Autodesk Fusion 360 part; units mm, degrees
(part 8 of 11)
  line L3162 (205.13, 80.0836) -> (204.329, 80.0836)
  line L3163 (43.205, 99.7592) -> (42.406, 99.7592)
  line L3164 (-9.983, 10.9337) -> (-9.183, 10.9337)
  line L3165 (247.333, 38.5083) -> (247.929, 38.5083)
  line L3166 (-9.183, 14.0343) -> (-9.983, 14.0343)
  line L3167 (-28.52, 61.0336) -> (-28.52, 62.034)
  line L3168 (252.529, 29.4092) -> (252.529, 30.2332)
  line L3169 (205.13, 71.1844) -> (205.13, 76.9844)
  line L3170 (-143.3331, 10.9337) -> (-143.3331, 14.0343)
  line L3171 (200.082, 80.0836) -> (200.879, 80.0836)
  line L3172 (204.329, 68.0838) -> (205.13, 68.0838)
  line L3173 (42.406, 105.5592) -> (42.406, 108.6602)
  line L3174 (-9.983, 10.9337) -> (-9.983, 14.0343)
  line L3175 (-114.244, 105.5592) -> (-113.445, 105.5592)
  line L3176 (-22.957, 33.0844) -> (-23.758, 33.0844)
  line L3177 (43.205, 108.6602) -> (43.205, 109.6602)
  line L3178 (256.681, 31.9583) -> (255.761, 31.9583)
  line L3179 (-140.9519, 0.7845) -> (-140.1512, 0.7845)
  line L3180 (-14.233, 10.9337) -> (-13.432, 10.9337)
  line L3181 (-140.1512, 0.7845) -> (-140.1512, -5.0157)
  line L3182 (-28.52, 48.0333) -> (-28.52, 49.0338)
  line L3183 (243.459, 30.2332) -> (249.732, 30.2332)
  line L3184 (-140.9519, -5.0157) -> (-140.9519, -8.1163)
  line L3185 (-23.758, 41.9836) -> (-23.758, 42.984)
  line L3186 (200.879, 80.0836) -> (200.879, 76.9844)
  line L3187 (-140.9519, 0.7845) -> (-140.9519, 3.8837)
  line L3188 (200.879, 68.0838) -> (200.082, 68.0838)
  line L3189 (-142.5325, 9.9333) -> (-142.5325, 10.9337)
  line L3190 (255.761, 31.9583) -> (255.761, 30.2332)
  line L3191 (249.732, 30.2332) -> (243.459, 30.2332)
  line L3192 (249.732, 30.2332) -> (249.732, 29.4092)
  line L3193 (205.13, 76.9844) -> (205.13, 71.1844)
  line L3194 (200.082, 81.084) -> (186.08, 81.084)
  line L3195 (200.082, 67.0833) -> (186.08, 67.0833)
  line L3196 (5.618, 10.9337) -> (4.817, 10.9337)
  line L3197 (-18.708, 41.9836) -> (-19.508, 41.9836)
  line L3198 (200.082, 71.1844) -> (200.879, 71.1844)
  line L3199 (7.398, -18.7426) -> (7.398, -15.9426)
  line L3200 (-140.9519, -5.0157) -> (-140.1512, -5.0157)
  line L3201 (-142.5325, 14.0343) -> (-143.3331, 14.0343)
  line L3202 (-143.3331, 14.0343) -> (-142.5325, 14.0343)
  line L3203 (43.205, 96.6592) -> (42.406, 96.6592)
  line L3204 (-27.72, 52.1344) -> (-28.52, 52.1344)
  line L3205 (-143.3331, 14.0343) -> (-143.3331, 10.9337)
  line L3206 (-143.3331, 10.9337) -> (-142.5325, 10.9337)
  line L3207 (4.817, 9.9333) -> (4.817, 10.9337)
  line L3208 (-18.708, 42.984) -> (-18.708, 41.9836)
  line L3209 (-18.708, 33.0844) -> (-19.508, 33.0844)
  line L3210 (9.581, 61.0336) -> (9.581, 62.034)
  line L3211 (-142.5325, 10.9337) -> (-143.3331, 10.9337)
  line L3212 (-13.432, 10.9337) -> (-14.233, 10.9337)
  line L3213 (-28.52, 61.0336) -> (-27.72, 61.0336)
  line L3214 (-18.708, 33.0844) -> (-18.708, 38.8844)
  line L3215 (4.817, 10.9337) -> (4.817, 9.9333)
  line L3216 (186.08, 81.084) -> (200.082, 81.084)
  line L3217 (42.406, 105.5592) -> (43.205, 105.5592)
  line L3218 (43.205, 96.6592) -> (43.205, 95.6582)
  line L3219 (-28.52, 52.1344) -> (-27.72, 52.1344)
  line L3220 (-27.72, 57.9344) -> (-28.52, 57.9344)
  line L3221 (-23.758, 33.0844) -> (-22.957, 33.0844)
  line L3222 (43.205, 109.6602) -> (43.205, 108.6602)
  line L3223 (186.08, 67.0833) -> (200.082, 67.0833)
  line L3224 (-114.758, 41.9836) -> (-114.758, 38.8844)
  line L3225 (-23.758, 38.8844) -> (-23.758, 33.0844)
  line L3226 (-140.9519, -8.1163) -> (-140.1512, -8.1163)
  line L3227 (-113.9576, 41.9836) -> (-114.758, 41.9836)
  line L3228 (9.867, 19.8345) -> (9.867, 14.0343)
  line L3229 (-44.901, 0.1836) -> (-84.5267, 0.1836)
  line L3230 (-28.52, 57.9344) -> (-27.72, 57.9344)
  line L3231 (28.798, 120.9832) -> (9.398, 120.9832)
  line L3232 (43.205, 108.6602) -> (42.406, 108.6602)
  line L3233 (42.406, 96.6592) -> (42.406, 99.7592)
  line L3234 (238.182, 62.034) -> (224.18, 62.034)
  line L3235 (-19.508, 38.8844) -> (-19.508, 41.9836)
  line L3236 (-28.52, 48.0333) -> (-42.52, 48.0333)
  line L3237 (-137.77, 48.0333) -> (-137.77, 49.0338)
  line L3238 (10.38, 49.0338) -> (10.38, 52.1344)
  line L3239 (9.581, 57.9344) -> (9.581, 52.1344)
  line L3240 (-13.432, 14.0343) -> (-13.432, 10.9337)
  line L3241 (-9.183, 9.9333) -> (-9.183, 10.9337)
  line L3242 (-9.183, 10.9337) -> (-9.983, 10.9337)
  line L3243 (14.63, 57.9344) -> (14.63, 52.1344)
  line L3244 (-14.233, 9.9333) -> (-14.233, 10.9337)
  line L3245 (-22.957, 41.9836) -> (-22.957, 38.8844)
  line L3246 (-23.758, 38.8844) -> (-22.957, 38.8844)
  line L3247 (-66.333, 23.934) -> (-52.333, 23.934)
  line L3248 (-137.77, 57.9344) -> (-138.5693, 57.9344)
  line L3249 (242.482, 55.7585) -> (242.482, 59.0591)
  line L3250 (-118.2075, 38.8844) -> (-118.2075, 41.9836)
  line L3251 (-42.52, 48.0333) -> (-28.52, 48.0333)
  line L3252 (-140.1512, 0.7845) -> (-140.9519, 0.7845)
  line L3253 (-23.758, 33.0844) -> (-23.758, 38.8844)
  line L3254 (-113.9576, 42.984) -> (-113.9576, 41.9836)
  line L3255 (-114.758, 33.0844) -> (-113.9576, 33.0844)
  line L3256 (43.205, 95.6582) -> (43.205, 96.6592)
  line L3257 (-138.5693, 57.9344) -> (-138.5693, 61.0336)
  line L3258 (19.106, 81.084) -> (5.105, 81.084)
  arc A55 (7.398, -18.7426) -> (9.398, -20.7426) centre (9.398, -18.7426) ccw
  line L3259 (-137.77, 62.034) -> (-137.77, 61.0336)
  line L3260 (-18.708, 38.8844) -> (-18.708, 33.0844)
  line L3261 (-149.9629, 14.0343) -> (-149.9629, 19.8345)
  line L3262 (-42.52, 62.034) -> (-28.52, 62.034)
  line L3263 (42.406, 99.7592) -> (42.406, 96.6592)
  line L3264 (-114.758, 38.8844) -> (-114.758, 41.9836)
  line L3265 (-57.094, 99.7592) -> (-57.094, 105.5592)
  line L3266 (42.406, 99.7592) -> (43.205, 99.7592)
  line L3267 (-138.5693, 57.9344) -> (-137.77, 57.9344)
  line L3268 (255.761, 60.7841) -> (252.529, 60.7841)
  line L3269 (-27.72, 49.0338) -> (-28.52, 49.0338)
  line L3270 (-19.508, 38.8844) -> (-18.708, 38.8844)
  line L3271 (9.398, -20.7426) -> (28.798, -20.7426)
  line L3272 (-138.5693, 52.1344) -> (-137.77, 52.1344)
  line L3273 (249.732, 61.6082) -> (249.732, 60.7841)
  line L3274 (-56.295, 99.7592) -> (-57.094, 99.7592)
  line L3275 (-113.9576, 33.0844) -> (-114.758, 33.0844)
  line L3276 (9.867, 9.9333) -> (23.867, 9.9333)
  line L3277 (-56.295, 96.6592) -> (-56.295, 99.7592)
  line L3278 (-118.2075, 41.9836) -> (-118.2075, 38.8844)
  line L3279 (43.205, 99.7592) -> (43.205, 105.5592)
  line L3280 (-27.72, 61.0336) -> (-28.52, 61.0336)
  line L3281 (249.732, 60.7841) -> (243.459, 60.7841)
  line L3282 (4.817, 14.0343) -> (4.817, 19.8345)
  line L3283 (-23.758, 42.984) -> (-23.758, 41.9836)
  line L3284 (42.406, 108.6602) -> (42.406, 105.5592)
  line L3285 (-28.52, 62.034) -> (-42.52, 62.034)
  line L3286 (-19.508, 41.9836) -> (-19.508, 38.8844)
  line L3287 (-137.77, 52.1344) -> (-137.77, 57.9344)
  line L3288 (238.182, 22.9336) -> (238.182, 23.934)
  line L3289 (238.182, 61.0336) -> (238.182, 62.034)
  line L3290 (23.867, 14.0343) -> (23.867, 19.8345)
  line L3291 (23.867, 9.9333) -> (9.867, 9.9333)
  line L3292 (43.205, 105.5592) -> (43.205, 99.7592)
  line L3293 (-28.52, 49.0338) -> (-27.72, 49.0338)
  line L3294 (-22.957, 38.8844) -> (-22.957, 41.9836)
  line L3295 (-114.244, 95.6582) -> (-128.2451, 95.6582)
  line L3296 (-19.508, 33.0844) -> (-18.708, 33.0844)
  line L3297 (-28.52, 57.9344) -> (-28.52, 52.1344)
  line L3298 (-57.094, 108.6602) -> (-56.295, 108.6602)
  line L3299 (-137.77, 61.0336) -> (-138.5693, 61.0336)
  line L3300 (-19.508, 41.9836) -> (-18.708, 41.9836)
  line L3301 (-57.094, 108.6602) -> (-57.094, 109.6602)
  line L3302 (-113.9576, 29.9838) -> (-113.9576, 28.9833)
  line L3303 (-137.77, 49.0338) -> (-138.5693, 49.0338)
  line L3304 (28.917, 19.8345) -> (28.917, 14.0343)
  line L3305 (-57.094, 95.6582) -> (-57.094, 96.6592)
  line L3306 (-14.233, 14.0343) -> (-14.233, 19.8345)
  line L3307 (-57.094, 96.6592) -> (-57.094, 95.6582)
  line L3308 (242.482, 20.959) -> (243.459, 20.959)
  line L3309 (43.205, 105.5592) -> (42.406, 105.5592)
  line L3310 (-56.295, 105.5592) -> (-57.094, 105.5592)
  line L3311 (-28.52, 52.1344) -> (-28.52, 57.9344)
  line L3312 (-22.957, 41.9836) -> (-23.758, 41.9836)
  line L3313 (-22.957, 38.8844) -> (-23.758, 38.8844)
  line L3314 (242.482, 59.0591) -> (243.459, 59.0591)
  line L3315 (42.406, 108.6602) -> (43.205, 108.6602)
  line L3316 (256.681, 59.0591) -> (255.761, 59.0591)
  line L3317 (-52.045, 67.0833) -> (-38.044, 67.0833)
  line L3318 (252.529, 22.6841) -> (255.761, 22.6841)
  line L3319 (-118.2075, 33.0844) -> (-118.2075, 29.9838)
  line L3320 (-113.9576, 29.9838) -> (-114.758, 29.9838)
  line L3321 (-137.77, 57.9344) -> (-137.77, 52.1344)
  line L3322 (238.979, 57.9344) -> (238.182, 57.9344)
  line L3323 (-14.233, 19.8345) -> (-14.233, 14.0343)
  line L3324 (243.459, 22.6841) -> (249.732, 22.6841)
  line L3325 (-114.758, 29.9838) -> (-114.758, 33.0844)
  line L3326 (-28.52, 62.034) -> (-28.52, 61.0336)
  line L3327 (-138.5693, 52.1344) -> (-138.5693, 49.0338)
  line L3328 (238.979, 61.0336) -> (238.979, 57.9344)
  line L3329 (-137.77, 61.0336) -> (-137.77, 62.034)
  line L3330 (4.817, 19.8345) -> (4.817, 14.0343)
  line L3331 (-114.758, 33.0844) -> (-114.758, 29.9838)
  line L3332 (-138.5693, 49.0338) -> (-138.5693, 52.1344)
  line L3333 (252.529, 60.7841) -> (252.529, 61.6082)
  line L3334 (-18.708, 41.9836) -> (-18.708, 42.984)
  line L3335 (249.732, 22.6841) -> (243.459, 22.6841)
  line L3336 (-143.2635, 114.1832) -> (-108.601, 114.1832)
  line L3337 (-57.094, 109.6602) -> (-57.094, 108.6602)
  line L3338 (-9.183, 14.0343) -> (-9.183, 19.8345)
  line L3339 (-163.9637, 19.8345) -> (-163.9637, 14.0343)
  line L3340 (-56.295, 105.5592) -> (-56.295, 108.6602)
  line L3341 (-113.9576, 38.8844) -> (-114.758, 38.8844)
  line L3342 (-137.77, 49.0338) -> (-137.77, 48.0333)
  line L3343 (28.917, 14.0343) -> (28.917, 19.8345)
  line L3344 (238.979, 19.8345) -> (238.182, 19.8345)
  line L3345 (-57.094, 105.5592) -> (-56.295, 105.5592)
  line L3346 (-149.9629, 9.9333) -> (-149.9629, 10.9337)
  line L3347 (42.917, 19.8345) -> (42.917, 14.0343)
  line L3348 (-114.758, 41.9836) -> (-113.9576, 41.9836)
  line L3349 (-9.183, 19.8345) -> (-9.183, 14.0343)
  line L3350 (249.732, 60.7841) -> (249.732, 61.6082)
  line L3351 (-23.758, 41.9836) -> (-22.957, 41.9836)
  line L3352 (-113.9576, 41.9836) -> (-113.9576, 42.984)
  line L3353 (-18.708, 38.8844) -> (-19.508, 38.8844)
  line L3354 (238.182, 19.8345) -> (238.979, 19.8345)
  line L3355 (238.182, 57.9344) -> (238.979, 57.9344)
  line L3356 (-57.094, 105.5592) -> (-57.094, 99.7592)
  line L3357 (-163.9637, 9.9333) -> (-163.9637, 10.9337)
  line L3358 (-138.5693, 61.0336) -> (-138.5693, 57.9344)
  line L3359 (-138.5693, 49.0338) -> (-137.77, 49.0338)
  line L3360 (9.867, 14.0343) -> (9.867, 19.8345)
  line L3361 (256.681, 20.959) -> (256.681, 17.6585)
  line L3362 (14.63, 49.0338) -> (13.831, 49.0338)
  line L3363 (252.529, 60.7841) -> (255.761, 60.7841)
  line L3364 (-118.2075, 29.9838) -> (-118.2075, 33.0844)
  line L3365 (238.182, 22.9336) -> (238.979, 22.9336)
  line L3366 (-57.094, 96.6592) -> (-56.295, 96.6592)
  line L3367 (-163.9637, 3.8837) -> (-163.9637, 4.8841)
  line L3368 (255.761, 20.959) -> (256.681, 20.959)
  line L3369 (-164.763, 14.0343) -> (-163.9637, 14.0343)
  line L3370 (42.917, 14.0343) -> (42.917, 19.8345)
  line L3371 (-138.5693, 61.0336) -> (-137.77, 61.0336)
  line L3372 (255.761, 20.959) -> (255.761, 22.6841)
  line L3373 (-56.295, 99.7592) -> (-56.295, 96.6592)
  line L3374 (255.761, 59.0591) -> (255.761, 60.7841)
  line L3375 (9.581, 52.1344) -> (10.38, 52.1344)
  line L3376 (-114.758, 29.9838) -> (-113.9576, 29.9838)
  line L3377 (-137.77, 52.1344) -> (-138.5693, 52.1344)
  line L3378 (-114.758, 38.8844) -> (-113.9576, 38.8844)
  line L3379 (243.459, 60.7841) -> (249.732, 60.7841)
  line L3380 (255.761, 59.0591) -> (256.681, 59.0591)
  line L3381 (-113.9576, 38.8844) -> (-113.9576, 33.0844)
  line L3382 (-163.9637, 4.8841) -> (-163.9637, 3.8837)
  line L3383 (-56.295, 108.6602) -> (-56.295, 105.5592)
  line L3384 (-142.5325, 14.0343) -> (-142.5325, 19.8345)
  line L3385 (10.38, 61.0336) -> (9.581, 61.0336)
  line L3386 (-29.033, 19.8345) -> (-28.233, 19.8345)
  line L3387 (13.831, 49.0338) -> (14.63, 49.0338)
  line L3388 (-56.295, 108.6602) -> (-57.094, 108.6602)
  line L3389 (255.761, 22.6841) -> (255.761, 20.959)
  line L3390 (-119.0079, 29.9838) -> (-118.2075, 29.9838)
  line L3391 (13.831, 52.1344) -> (13.831, 49.0338)
  line L3392 (-118.2075, 33.0844) -> (-119.0079, 33.0844)
  line L3393 (-164.763, 3.8837) -> (-163.9637, 3.8837)
  line L3394 (242.482, 59.0591) -> (242.482, 55.7585)
  line L3395 (-56.295, 96.6592) -> (-57.094, 96.6592)
  line L3396 (243.459, 59.0591) -> (242.482, 59.0591)
  line L3397 (13.831, 99.7592) -> (13.831, 96.6592)
  line L3398 (-113.9576, 28.9833) -> (-113.9576, 29.9838)
  line L3399 (14.63, 99.7592) -> (13.831, 99.7592)
  line L3400 (-57.094, 99.7592) -> (-56.295, 99.7592)
  line L3401 (242.482, 20.959) -> (242.482, 17.6585)
  line L3402 (-149.9629, 3.8837) -> (-149.1636, 3.8837)
  line L3403 (238.182, 67.0833) -> (224.18, 67.0833)
  line L3404 (-32.995, 67.0833) -> (-32.995, 68.0838)
  line L3405 (-113.9576, 33.0844) -> (-113.9576, 38.8844)
  line L3406 (-164.763, 10.9337) -> (-163.9637, 10.9337)
  line L3407 (-163.9637, 9.9333) -> (-149.9629, 9.9333)
  line L3408 (243.459, 20.959) -> (243.459, 22.6841)
  line L3409 (242.482, 17.6585) -> (242.482, 20.959)
  line L3410 (-4.42, 95.6582) -> (9.581, 95.6582)
  line L3411 (-33.794, 80.0836) -> (-32.995, 80.0836)
  line L3412 (238.979, 57.9344) -> (238.979, 61.0336)
  line L3413 (-33.794, 76.9844) -> (-33.794, 80.0836)
  line L3414 (252.529, 61.6082) -> (252.529, 60.7841)
  line L3415 (-28.233, 22.9336) -> (-29.033, 22.9336)
  line L3416 (9.581, 52.1344) -> (9.581, 57.9344)
  line L3417 (-32.995, 68.0838) -> (-32.995, 67.0833)
  line L3418 (28.631, 99.7592) -> (29.43, 99.7592)
  line L3419 (28.631, 96.6592) -> (29.43, 96.6592)
  line L3420 (256.681, 20.959) -> (255.761, 20.959)
  line L3421 (-33.794, 71.1844) -> (-32.995, 71.1844)
  line L3422 (238.182, 23.934) -> (238.182, 22.9336)
  line L3423 (9.581, 105.5592) -> (9.581, 99.7592)
  line L3424 (14.63, 61.0336) -> (14.63, 62.034)
  line L3425 (29.43, 96.6592) -> (28.631, 96.6592)
  line L3426 (-118.2075, 29.9838) -> (-119.0079, 29.9838)
  line L3427 (-32.995, 76.9844) -> (-32.995, 71.1844)
  line L3428 (-119.0079, 41.9836) -> (-119.0079, 42.984)
  line L3429 (14.63, 96.6592) -> (14.63, 95.6582)
  line L3430 (249.732, 22.6841) -> (249.732, 23.5082)
  line L3431 (-119.0079, 38.8844) -> (-119.0079, 33.0844)
  line L3432 (-163.9637, 10.9337) -> (-163.9637, 9.9333)
  line L3433 (-149.9629, 14.0343) -> (-149.1636, 14.0343)
  line L3434 (10.38, 61.0336) -> (10.38, 57.9344)
  line L3435 (243.459, 59.0591) -> (243.459, 60.7841)
  line L3436 (238.182, 62.034) -> (238.182, 61.0336)
  line L3437 (-33.794, 68.0838) -> (-33.794, 71.1844)
  line L3438 (9.581, 96.6592) -> (9.581, 95.6582)
  line L3439 (-149.9629, 3.8837) -> (-149.9629, 4.8841)
  line L3440 (-28.233, 19.8345) -> (-29.033, 19.8345)
  line L3441 (-33.794, 76.9844) -> (-32.995, 76.9844)
  line L3442 (-18.708, 29.9838) -> (-18.708, 28.9833)
  line L3443 (-71.8941, 96.6592) -> (-71.8941, 99.7592)
  line L3444 (-71.8941, 108.6602) -> (-71.8941, 105.5592)
  line L3445 (255.761, 22.6841) -> (252.529, 22.6841)
  line L3446 (-71.8941, 99.7592) -> (-71.8941, 96.6592)
  line L3447 (-149.1636, 3.8837) -> (-149.9629, 3.8837)
  line L3448 (252.529, 61.6082) -> (249.732, 61.6082)
  line L3449 (243.459, 60.7841) -> (243.459, 59.0591)
  line L3450 (-23.758, 29.9838) -> (-22.957, 29.9838)
  line L3451 (14.63, 57.9344) -> (13.831, 57.9344)
  line L3452 (13.831, 96.6592) -> (14.63, 96.6592)
  line L3453 (-118.2075, 38.8844) -> (-119.0079, 38.8844)
  line L3454 (10.38, 99.7592) -> (9.581, 99.7592)
  line L3455 (14.63, 61.0336) -> (13.831, 61.0336)
  line L3456 (14.63, 95.6582) -> (14.63, 96.6592)
  line L3457 (-23.758, 28.9833) -> (-23.758, 29.9838)
  line L3458 (-33.794, 80.0836) -> (-33.794, 76.9844)
  line L3459 (-71.8941, 105.5592) -> (-71.8941, 108.6602)
  line L3460 (249.732, 23.5082) -> (249.732, 22.6841)
  line L3461 (-29.033, 22.9336) -> (-29.033, 19.8345)
  line L3462 (-28.233, 22.9336) -> (-28.233, 23.934)
  line L3463 (29.43, 99.7592) -> (29.43, 96.6592)
  line L3464 (-164.763, 14.0343) -> (-164.763, 10.9337)
  line L3465 (28.631, 96.6592) -> (28.631, 95.6582)
  line L3466 (238.979, 61.0336) -> (238.182, 61.0336)
  line L3467 (-32.995, 80.0836) -> (-32.995, 81.084)
  line L3468 (-57.094, 109.6602) -> (-71.095, 109.6602)
  line L3469 (9.581, 109.6602) -> (9.581, 108.6602)
  line L3470 (-75.345, 108.6602) -> (-76.144, 108.6602)
  line L3471 (13.831, 49.0338) -> (13.831, 52.1344)
  line L3472 (-149.1636, 10.9337) -> (-149.9629, 10.9337)
  line L3473 (9.581, 108.6602) -> (10.38, 108.6602)
  line L3474 (-149.9629, 4.8841) -> (-149.9629, 3.8837)
  line L3475 (238.979, 22.9336) -> (238.979, 19.8345)
  line L3476 (256.681, 55.7585) -> (256.681, 59.0591)
  line L3477 (243.459, 22.6841) -> (243.459, 20.959)
  line L3478 (-119.0079, 28.9833) -> (-119.0079, 29.9838)
  line L3479 (-71.8941, 108.6602) -> (-71.095, 108.6602)
  line L3480 (-32.995, 81.084) -> (-32.995, 80.0836)
  line L3481 (-119.0079, 33.0844) -> (-119.0079, 38.8844)
  line L3482 (255.761, 60.7841) -> (255.761, 59.0591)
  line L3483 (14.63, 62.034) -> (14.63, 61.0336)
  line L3484 (-119.0079, 42.984) -> (-119.0079, 41.9836)
  line L3485 (-163.9637, 3.8837) -> (-164.763, 3.8837)
  line L3486 (-71.8941, 99.7592) -> (-71.095, 99.7592)
  line L3487 (-33.794, 68.0838) -> (-32.995, 68.0838)
  line L3488 (-83.201, 118.9832) -> (-83.201, 116.1832)
  line L3489 (-119.0079, 38.8844) -> (-118.2075, 38.8844)
  line L3490 (-32.995, 68.0838) -> (-33.794, 68.0838)
  line L3491 (9.581, 49.0338) -> (9.581, 48.0333)
  line L3492 (10.38, 96.6592) -> (10.38, 99.7592)
  line L3493 (-32.995, 80.0836) -> (-33.794, 80.0836)
  line L3494 (-71.095, 105.5592) -> (-71.8941, 105.5592)
  line L3495 (256.681, 59.0591) -> (256.681, 55.7585)
  line L3496 (238.979, 22.9336) -> (238.182, 22.9336)
  line L3497 (-22.957, 29.9838) -> (-23.758, 29.9838)
  line L3498 (9.581, 99.7592) -> (9.581, 105.5592)
  line L3499 (-71.095, 109.6602) -> (-71.095, 108.6602)
  line L3500 (-75.345, 99.7592) -> (-76.144, 99.7592)
  line L3501 (-119.0079, 29.9838) -> (-119.0079, 28.9833)
  line L3502 (10.38, 57.9344) -> (10.38, 61.0336)
  line L3503 (249.732, 61.6082) -> (252.529, 61.6082)
  line L3504 (-119.0079, 33.0844) -> (-118.2075, 33.0844)
  line L3505 (-76.144, 99.7592) -> (-75.345, 99.7592)
  line L3506 (14.63, 95.6582) -> (28.631, 95.6582)
  line L3507 (28.631, 95.6582) -> (14.63, 95.6582)
  line L3508 (10.38, 96.6592) -> (9.581, 96.6592)
  line L3509 (-18.708, 29.9838) -> (-19.508, 29.9838)
  line L3510 (-163.9637, 4.8841) -> (-149.9629, 4.8841)
  line L3511 (28.631, 95.6582) -> (28.631, 96.6592)
  line L3512 (-23.758, 29.9838) -> (-23.758, 28.9833)
  line L3513 (249.732, 23.5082) -> (252.529, 23.5082)
  line L3514 (-149.9629, 4.8841) -> (-163.9637, 4.8841)
  line L3515 (-128.2451, 71.1844) -> (-129.0441, 71.1844)
  line L3516 (-29.033, 22.9336) -> (-28.233, 22.9336)
  line L3517 (238.979, 19.8345) -> (238.979, 22.9336)
  line L3518 (-32.995, 71.1844) -> (-33.794, 71.1844)
  line L3519 (-118.2075, 41.9836) -> (-119.0079, 41.9836)
  line L3520 (-132.495, 76.9844) -> (-133.294, 76.9844)
  line L3521 (252.529, 22.6841) -> (252.529, 23.5082)
  line L3522 (-32.995, 71.1844) -> (-32.995, 76.9844)
  line L3523 (-32.995, 76.9844) -> (-33.794, 76.9844)
  line L3524 (-132.495, 68.0838) -> (-133.294, 68.0838)
  line L3525 (-71.095, 96.6592) -> (-71.8941, 96.6592)
  line L3526 (10.38, 99.7592) -> (10.38, 96.6592)
  line L3527 (-28.233, 23.934) -> (-28.233, 22.9336)
  line L3528 (13.831, 99.7592) -> (14.63, 99.7592)
  arc A56 (9.398, 120.9832) -> (7.398, 118.9832) centre (9.398, 118.9832) ccw
  line L3529 (-76.144, 105.5592) -> (-76.144, 99.7592)
  line L3530 (-71.8941, 96.6592) -> (-71.095, 96.6592)
  line L3531 (13.831, 96.6592) -> (13.831, 99.7592)
  line L3532 (238.182, 61.0336) -> (238.979, 61.0336)
  line L3533 (9.581, 105.5592) -> (10.38, 105.5592)
  line L3534 (-19.508, 29.9838) -> (-18.708, 29.9838)
  line L3535 (9.581, 108.6602) -> (9.581, 109.6602)
  line L3536 (29.43, 99.7592) -> (28.631, 99.7592)
  line L3537 (-132.495, 80.0836) -> (-132.495, 76.9844)
  line L3538 (-76.144, 108.6602) -> (-75.345, 108.6602)
  line L3539 (-76.144, 96.6592) -> (-76.144, 95.6582)
  line L3540 (-18.708, 28.9833) -> (-18.708, 29.9838)
  line L3541 (-149.1636, 14.0343) -> (-149.9629, 14.0343)
  line L3542 (-149.9629, 9.9333) -> (-163.9637, 9.9333)
  line L3543 (-149.1636, 10.9337) -> (-149.1636, 14.0343)
  line L3544 (-71.095, 95.6582) -> (-57.094, 95.6582)
  line L3545 (-119.0079, 41.9836) -> (-118.2075, 41.9836)
  line L3546 (256.681, 17.6585) -> (256.681, 20.959)
  line L3547 (29.43, 96.6592) -> (29.43, 99.7592)
  line L3548 (-147.583, 57.9344) -> (-147.583, 52.1344)
  line L3549 (-5.219, 49.0338) -> (-5.219, 52.1344)
  line L3550 (-42.007, 29.9838) -> (-42.007, 33.0844)
  line L3551 (256.23, 15.2084) -> (256.23, 14.4091)
  line L3552 (-42.808, 41.9836) -> (-42.007, 41.9836)
  line L3553 (-9.469, 109.6602) -> (-9.469, 108.6602)
  line L3554 (-104.4326, 9.9333) -> (-104.4326, 10.9337)
  line L3555 (-8.67, 49.0338) -> (-8.67, 52.1344)
  line L3556 (-9.469, 49.0338) -> (-9.469, 48.0333)
  line L3557 (247.929, -1.1159) -> (243.459, -1.1159)
  line L3558 (238.182, -9.1167) -> (238.182, -8.1163)
  line L3559 (253.129, 14.4091) -> (252.529, 14.4091)
  line L3560 (-8.67, 108.6602) -> (-9.469, 108.6602)
  line L3561 (-4.42, 57.9344) -> (-4.42, 52.1344)
  line L3562 (-4.42, 61.0336) -> (-5.219, 61.0336)
  line L3563 (-105.233, 10.9337) -> (-104.4326, 10.9337)
  line L3564 (255.761, 17.6585) -> (256.681, 17.6585)
  line L3565 (-9.469, 108.6602) -> (-8.67, 108.6602)
  line L3566 (-9.469, 99.7592) -> (-9.469, 105.5592)
  line L3567 (-4.42, 109.6602) -> (9.581, 109.6602)
  line L3568 (249.732, -7.8669) -> (243.459, -7.8669)
  line L3569 (243.459, -7.8669) -> (249.732, -7.8669)
  line L3570 (-61.57, 52.1344) -> (-62.371, 52.1344)
  line L3571 (238.979, 0.7845) -> (238.979, 3.8837)
  line L3572 (-37.758, 33.0844) -> (-37.758, 38.8844)
  line L3573 (-9.469, 49.0338) -> (-8.67, 49.0338)
  line L3574 (-147.583, 61.0336) -> (-147.583, 62.034)
  line L3575 (-4.42, 62.034) -> (-4.42, 61.0336)
  line L3576 (-37.758, 29.9838) -> (-37.758, 28.9833)
  line L3577 (252.529, 15.9333) -> (252.529, 14.4091)
  line L3578 (-8.67, 52.1344) -> (-9.469, 52.1344)
  line L3579 (-147.583, 49.0338) -> (-146.7824, 49.0338)
  line L3580 (0.855, 80.0836) -> (0.056, 80.0836)
  line L3581 (255.761, 15.9333) -> (255.761, 17.6585)
  line L3582 (-9.469, 96.6592) -> (-8.67, 96.6592)
  line L3583 (-105.233, 14.0343) -> (-105.233, 10.9337)
  line L3584 (-8.67, 52.1344) -> (-8.67, 49.0338)
  line L3585 (238.182, -8.1163) -> (238.979, -8.1163)
  line L3586 (-146.7824, 49.0338) -> (-147.583, 49.0338)
  line L3587 (-5.219, 52.1344) -> (-4.42, 52.1344)
  line L3588 (-42.808, 29.9838) -> (-42.007, 29.9838)
  line L3589 (252.529, 14.4091) -> (252.529, 15.9333)
  line L3590 (-4.42, 57.9344) -> (-5.219, 57.9344)
  line L3591 (-8.67, 61.0336) -> (-8.67, 57.9344)
  line L3592 (-104.4326, 14.0343) -> (-104.4326, 19.8345)
  line L3593 (-42.808, 38.8844) -> (-42.007, 38.8844)
  line L3594 (-147.583, 49.0338) -> (-147.583, 48.0333)
  line L3595 (-129.0441, 105.5592) -> (-128.2451, 105.5592)
  line L3596 (253.129, 14.4091) -> (253.129, 15.2084)
  line L3597 (255.761, 17.6585) -> (255.761, 15.9333)
  line L3598 (4.306, 71.1844) -> (4.306, 68.0838)
  line L3599 (-9.469, 48.0333) -> (-9.469, 49.0338)
  line L3600 (238.182, 3.8837) -> (238.182, 4.8841)
  line L3601 (-9.469, 95.6582) -> (-9.469, 96.6592)
  line L3602 (238.182, 0.7845) -> (238.979, 0.7845)
  line L3603 (-104.4326, 10.9337) -> (-104.4326, 9.9333)
  line L3604 (-8.67, 99.7592) -> (-9.469, 99.7592)
  line L3605 (-42.808, 41.9836) -> (-42.808, 42.984)
  line L3606 (-109.4829, 19.8345) -> (-109.4829, 14.0343)
  line L3607 (-56.808, 28.9833) -> (-42.808, 28.9833)
  line L3608 (4.306, 76.9844) -> (4.306, 80.0836)
  line L3609 (-89.6325, 10.9337) -> (-90.4329, 10.9337)
  line L3610 (-8.67, 49.0338) -> (-9.469, 49.0338)
  line L3611 (-146.7824, 57.9344) -> (-147.583, 57.9344)
  line L3612 (-71.095, 99.7592) -> (-71.8941, 99.7592)
  line L3613 (-33.794, 71.1844) -> (-33.794, 68.0838)
  line L3614 (252.529, 23.5082) -> (252.529, 22.6841)
  line L3615 (-149.9629, 10.9337) -> (-149.1636, 10.9337)
  line L3616 (-132.495, 71.1844) -> (-132.495, 68.0838)
  line L3617 (243.459, 20.959) -> (242.482, 20.959)
  line L3618 (-19.508, 29.9838) -> (-19.508, 33.0844)
  line L3619 (-129.0441, 80.0836) -> (-128.2451, 80.0836)
  line L3620 (14.63, 96.6592) -> (13.831, 96.6592)
  line L3621 (-75.345, 99.7592) -> (-75.345, 96.6592)
  line L3622 (-164.763, 10.9337) -> (-164.763, 14.0343)
  line L3623 (-76.144, 96.6592) -> (-75.345, 96.6592)
  line L3624 (-132.495, 68.0838) -> (-132.495, 71.1844)
  line L3625 (-57.094, 95.6582) -> (-71.095, 95.6582)
  line L3626 (-19.508, 33.0844) -> (-19.508, 29.9838)
  line L3627 (-163.9637, 14.0343) -> (-164.763, 14.0343)
  line L3628 (-22.957, 29.9838) -> (-22.957, 33.0844)
  line L3629 (-133.294, 76.9844) -> (-132.495, 76.9844)
  arc A57 (5.398, 114.1832) -> (7.398, 116.1832) centre (5.398, 116.1832) ccw
  line L3630 (10.38, 105.5592) -> (9.581, 105.5592)
  line L3631 (9.581, 99.7592) -> (10.38, 99.7592)
  line L3632 (-128.2451, 81.084) -> (-128.2451, 80.0836)
  line L3633 (-71.095, 99.7592) -> (-71.095, 105.5592)
  line L3634 (-76.144, 95.6582) -> (-76.144, 96.6592)
  line L3635 (-76.144, 99.7592) -> (-76.144, 105.5592)
  line L3636 (7.398, 118.9832) -> (7.398, 116.1832)
  line L3637 (252.529, 23.5082) -> (249.732, 23.5082)
  line L3638 (-29.033, 19.8345) -> (-29.033, 22.9336)
  line L3639 (-163.9637, 10.9337) -> (-164.763, 10.9337)
  line L3640 (-71.095, 109.6602) -> (-57.094, 109.6602)
  line L3641 (10.38, 108.6602) -> (10.38, 105.5592)
  line L3642 (-76.144, 105.5592) -> (-75.345, 105.5592)
  line L3643 (-71.095, 108.6602) -> (-71.8941, 108.6602)
  line L3644 (19.905, 80.0836) -> (19.106, 80.0836)
  line L3645 (-75.345, 105.5592) -> (-76.144, 105.5592)
  line L3646 (-76.144, 109.6602) -> (-76.144, 108.6602)
  line L3647 (19.106, 80.0836) -> (19.905, 80.0836)
  line L3648 (10.38, 105.5592) -> (10.38, 108.6602)
  line L3649 (-71.8941, 105.5592) -> (-71.095, 105.5592)
  line L3650 (-129.0441, 68.0838) -> (-129.0441, 71.1844)
  line L3651 (242.429, 68.0838) -> (243.23, 68.0838)
  line L3652 (-149.9629, 10.9337) -> (-149.9629, 9.9333)
  line L3653 (-71.095, 95.6582) -> (-71.095, 96.6592)
  line L3654 (19.905, 71.1844) -> (19.106, 71.1844)
  line L3655 (19.106, 67.0833) -> (19.106, 68.0838)
  line L3656 (-133.294, 68.0838) -> (-133.294, 67.0833)
  line L3657 (-22.957, 33.0844) -> (-22.957, 29.9838)
  line L3658 (-75.345, 105.5592) -> (-75.345, 108.6602)
  line L3659 (238.182, 68.0838) -> (238.979, 68.0838)
  line L3660 (-129.0441, 71.1844) -> (-128.2451, 71.1844)
  line L3661 (-37.245, 76.9844) -> (-37.245, 80.0836)
  line L3662 (-75.345, 96.6592) -> (-76.144, 96.6592)
  line L3663 (-71.095, 105.5592) -> (-71.095, 99.7592)
  line L3664 (-38.044, 71.1844) -> (-38.044, 76.9844)
  line L3665 (-71.095, 96.6592) -> (-71.095, 95.6582)
  line L3666 (9.581, 96.6592) -> (10.38, 96.6592)
  line L3667 (9.581, 95.6582) -> (9.581, 96.6592)
  line L3668 (10.38, 108.6602) -> (9.581, 108.6602)
  line L3669 (-71.095, 108.6602) -> (-71.095, 109.6602)
  line L3670 (19.905, 68.0838) -> (19.905, 71.1844)
  line L3671 (238.979, 71.1844) -> (238.979, 68.0838)
  line L3672 (-133.294, 80.0836) -> (-133.294, 81.084)
  line L3673 (-149.1636, 14.0343) -> (-149.1636, 10.9337)
  line L3674 (-76.144, 108.6602) -> (-76.144, 109.6602)
  line L3675 (-132.495, 80.0836) -> (-133.294, 80.0836)
  line L3676 (258.029, 68.0838) -> (257.232, 68.0838)
  line L3677 (-128.5329, 19.8345) -> (-127.7325, 19.8345)
  line L3678 (-75.345, 108.6602) -> (-75.345, 105.5592)
  line L3679 (258.029, 68.0838) -> (258.029, 71.1844)
  line L3680 (-128.2451, 80.0836) -> (-129.0441, 80.0836)
  line L3681 (5.105, 67.0833) -> (19.106, 67.0833)
  line L3682 (-4.42, 48.0333) -> (9.581, 48.0333)
  line L3683 (257.232, 68.0838) -> (258.029, 68.0838)
  line L3684 (-38.044, 68.0838) -> (-37.245, 68.0838)
  line L3685 (-38.044, 71.1844) -> (-37.245, 71.1844)
  line L3686 (238.182, 42.984) -> (224.18, 42.984)
  line L3687 (-42.808, 28.9833) -> (-56.808, 28.9833)
  line L3688 (-38.044, 67.0833) -> (-38.044, 68.0838)
  line L3689 (19.106, 76.9844) -> (19.106, 71.1844)
  line L3690 (19.106, 68.0838) -> (19.905, 68.0838)
  line L3691 (-123.4826, 22.9336) -> (-124.283, 22.9336)
  arc A58 (-83.201, 116.1832) -> (-81.201, 114.1832) centre (-81.201, 116.1832) ccw
  line L3692 (19.106, 80.0836) -> (19.106, 81.084)
  line L3693 (224.18, 67.0833) -> (238.182, 67.0833)
  arc A59 (-83.201, 118.9832) -> (-85.201, 120.9832) centre (-85.201, 118.9832) ccw
  line L3694 (-38.044, 80.0836) -> (-38.044, 81.084)
  line L3695 (-129.0441, 76.9844) -> (-129.0441, 80.0836)
  line L3696 (243.23, 68.0838) -> (242.429, 68.0838)
  line L3697 (-38.044, 80.0836) -> (-37.245, 80.0836)
  line L3698 (-75.345, 96.6592) -> (-75.345, 99.7592)
  line L3699 (238.979, 71.1844) -> (238.182, 71.1844)
  line L3700 (19.905, 76.9844) -> (19.106, 76.9844)
  line L3701 (-4.42, 62.034) -> (9.581, 62.034)
  line L3702 (-37.245, 76.9844) -> (-38.044, 76.9844)
  line L3703 (-108.6825, 22.9336) -> (-109.4829, 22.9336)
  line L3704 (-104.4326, 19.8345) -> (-104.4326, 14.0343)
  line L3705 (19.106, 81.084) -> (19.106, 80.0836)
  line L3706 (14.63, 108.6602) -> (13.831, 108.6602)
  line L3707 (19.106, 76.9844) -> (19.905, 76.9844)
  line L3708 (243.23, 68.0838) -> (243.23, 67.0833)
  line L3709 (-128.5329, 22.9336) -> (-128.5329, 23.934)
  line L3710 (-133.294, 71.1844) -> (-132.495, 71.1844)
  line L3711 (-37.245, 68.0838) -> (-38.044, 68.0838)
  line L3712 (238.182, 67.0833) -> (238.182, 68.0838)
  line L3713 (28.631, 99.7592) -> (28.631, 105.5592)
  line L3714 (238.182, 71.1844) -> (238.979, 71.1844)
  line L3715 (13.831, 108.6602) -> (13.831, 105.5592)
  line L3716 (-149.1636, 0.7845) -> (-149.9629, 0.7845)
  line L3717 (-124.283, 22.9336) -> (-124.283, 19.8345)
  line L3718 (-38.044, 68.0838) -> (-38.044, 67.0833)
  circle A60 centre (19.098, 117.5832) radius 1.7
  line L3719 (-52.045, 81.084) -> (-38.044, 81.084)
  line L3720 (19.905, 76.9844) -> (19.905, 80.0836)
  line L3721 (247.333, 14.4091) -> (247.929, 14.4091)
  line L3722 (-149.9629, -9.1167) -> (-149.9629, -8.1163)
  line L3723 (-132.495, 76.9844) -> (-132.495, 80.0836)
  line L3724 (-133.294, 76.9844) -> (-133.294, 71.1844)
  line L3725 (-123.4826, 23.934) -> (-109.4829, 23.934)
  line L3726 (-123.769, 48.0333) -> (-137.77, 48.0333)
  line L3727 (247.333, 15.2084) -> (244.232, 15.2084)
  line L3728 (9.581, 62.034) -> (-4.42, 62.034)
  line L3729 (19.905, 71.1844) -> (19.905, 68.0838)
  line L3730 (238.979, 68.0838) -> (238.182, 68.0838)
  line L3731 (-128.5329, 22.9336) -> (-127.7325, 22.9336)
  line L3732 (224.18, 62.034) -> (238.182, 62.034)
  line L3733 (-37.245, 80.0836) -> (-38.044, 80.0836)
  line L3734 (19.106, 71.1844) -> (19.905, 71.1844)
  line L3735 (-129.0441, 80.0836) -> (-129.0441, 76.9844)
  line L3736 (28.631, 108.6602) -> (29.43, 108.6602)
  line L3737 (-109.4829, 23.934) -> (-123.4826, 23.934)
  line L3738 (-137.77, 48.0333) -> (-123.769, 48.0333)
  line L3739 (-164.763, -5.0157) -> (-164.763, -8.1163)
  line L3740 (19.905, 68.0838) -> (19.106, 68.0838)
  line L3741 (-38.558, 41.9836) -> (-38.558, 38.8844)
  line L3742 (-108.6825, 19.8345) -> (-108.6825, 22.9336)
  line L3743 (-137.77, 62.034) -> (-123.769, 62.034)
  line L3744 (19.106, 71.1844) -> (19.106, 76.9844)
  line L3745 (19.106, 68.0838) -> (19.106, 67.0833)
  line L3746 (9.581, 48.0333) -> (-4.42, 48.0333)
  line L3747 (-128.2451, 81.084) -> (-114.244, 81.084)
  line L3748 (257.232, 67.0833) -> (243.23, 67.0833)
  line L3749 (-37.245, 71.1844) -> (-38.044, 71.1844)
  line L3750 (28.631, 105.5592) -> (28.631, 99.7592)
  line L3751 (-42.007, 41.9836) -> (-42.007, 38.8844)
  line L3752 (-133.294, 81.084) -> (-133.294, 80.0836)
  line L3753 (19.905, 80.0836) -> (19.905, 76.9844)
  line L3754 (-38.044, 76.9844) -> (-38.044, 71.1844)
  line L3755 (257.232, 68.0838) -> (257.232, 67.0833)
  line L3756 (-149.9629, -5.0157) -> (-149.1636, -5.0157)
  line L3757 (243.23, 71.1844) -> (242.429, 71.1844)
  line L3758 (9.581, 95.6582) -> (-4.42, 95.6582)
  line L3759 (19.498, 120.9832) -> (18.698, 120.9832)
  line L3760 (-149.1636, -8.1163) -> (-149.1636, -5.0157)
  line L3761 (-37.245, 71.1844) -> (-37.245, 68.0838)
  line L3762 (-133.294, 67.0833) -> (-133.294, 68.0838)
  line L3763 (-149.9629, 0.7845) -> (-149.9629, -5.0157)
  line L3764 (-37.245, 68.0838) -> (-37.245, 71.1844)
  line L3765 (-123.4826, 14.0343) -> (-123.4826, 19.8345)
  arc A61 (30.798, 118.9832) -> (28.798, 120.9832) centre (28.798, 118.9832) ccw
  line L3766 (243.23, 67.0833) -> (257.232, 67.0833)
  line L3767 (-90.4329, 19.8345) -> (-90.4329, 14.0343)
  line L3768 (30.798, 118.9832) -> (30.798, 116.1832)
  line L3769 (-38.044, 76.9844) -> (-37.245, 76.9844)
  line L3770 (244.232, 14.4091) -> (243.23, 14.4091)
  line L3771 (-108.6825, 22.9336) -> (-108.6825, 19.8345)
  line L3772 (-128.2451, 76.9844) -> (-129.0441, 76.9844)
  line L3773 (-5.219, 96.6592) -> (-4.42, 96.6592)
  line L3774 (243.23, 14.4091) -> (244.232, 14.4091)
  line L3775 (-37.245, 80.0836) -> (-37.245, 76.9844)
  line L3776 (-149.9629, 0.7845) -> (-149.1636, 0.7845)
  line L3777 (29.43, 105.5592) -> (28.631, 105.5592)
  line L3778 (28.631, 48.0333) -> (14.63, 48.0333)
  line L3779 (-37.758, 28.9833) -> (-37.758, 29.9838)
  line L3780 (-84.5267, 0.1836) -> (-44.901, 0.1836)
  line L3781 (257.232, 71.1844) -> (258.029, 71.1844)
  line L3782 (-38.558, 29.9838) -> (-37.758, 29.9838)
  line L3783 (14.63, 48.0333) -> (28.631, 48.0333)
  line L3784 (257.232, 67.0833) -> (257.232, 68.0838)
  line L3785 (28.631, 109.6602) -> (28.631, 108.6602)
  line L3786 (-149.9629, -8.1163) -> (-149.9629, -9.1167)
  line L3787 (-142.5325, 19.8345) -> (-142.5325, 14.0343)
  line L3788 (-124.283, 19.8345) -> (-124.283, 22.9336)
  line L3789 (-132.495, 71.1844) -> (-133.294, 71.1844)
  line L3790 (14.63, 105.5592) -> (13.831, 105.5592)
  line L3791 (-128.5329, 19.8345) -> (-128.5329, 14.0343)
  line L3792 (-164.763, 0.7845) -> (-163.9637, 0.7845)
  line L3793 (-109.4829, 14.0343) -> (-109.4829, 19.8345)
  line L3794 (-133.294, 80.0836) -> (-132.495, 80.0836)
  line L3795 (-38.044, 81.084) -> (-38.044, 80.0836)
  line L3796 (-123.4826, 23.934) -> (-123.4826, 22.9336)
  line L3797 (5.105, 81.084) -> (19.106, 81.084)
  line L3798 (247.333, 14.4091) -> (247.333, 15.2084)
  line L3799 (-163.9637, 14.0343) -> (-163.9637, 19.8345)
  line L3800 (14.63, 109.6602) -> (28.631, 109.6602)
  line L3801 (247.929, 14.4091) -> (247.929, 15.9333)
  line L3802 (-164.763, -8.1163) -> (-163.9637, -8.1163)
  line L3803 (258.029, 71.1844) -> (257.232, 71.1844)
  line L3804 (-128.2451, 67.0833) -> (-128.2451, 68.0838)
  line L3805 (-109.4829, 19.8345) -> (-108.6825, 19.8345)
  line L3806 (242.429, 71.1844) -> (242.429, 68.0838)
  line L3807 (14.63, 62.034) -> (28.631, 62.034)
  line L3808 (-4.42, 99.7592) -> (-5.219, 99.7592)
  line L3809 (243.23, 67.0833) -> (243.23, 68.0838)
  line L3810 (-52.333, 23.934) -> (-66.333, 23.934)
  line L3811 (238.182, 10.9337) -> (238.182, 9.9333)
  line L3812 (28.631, 108.6602) -> (28.631, 109.6602)
  line L3813 (-149.1636, -5.0157) -> (-149.9629, -5.0157)
  line L3814 (-5.219, 96.6592) -> (-5.219, 99.7592)
  line L3815 (-129.0441, 68.0838) -> (-128.2451, 68.0838)
  line L3816 (-47.569, 48.0333) -> (-61.57, 48.0333)
  line L3817 (-127.7325, 22.9336) -> (-127.7325, 19.8345)
  line L3818 (-5.219, 99.7592) -> (-4.42, 99.7592)
  arc A62 (30.798, 116.1832) -> (32.798, 114.1832) centre (32.798, 116.1832) ccw
  line L3819 (247.333, 15.2084) -> (247.333, 14.4091)
  line L3820 (-129.0441, 71.1844) -> (-129.0441, 68.0838)
  line L3821 (-4.42, 105.5592) -> (-4.42, 99.7592)
  line L3822 (-163.9637, -8.1163) -> (-163.9637, -9.1167)
  line L3823 (28.631, 62.034) -> (14.63, 62.034)
  line L3824 (-123.4826, 19.8345) -> (-124.283, 19.8345)
  line L3825 (-109.4829, 22.9336) -> (-108.6825, 22.9336)
  line L3826 (-163.9637, -8.1163) -> (-164.763, -8.1163)
  line L3827 (242.429, 68.0838) -> (242.429, 71.1844)
  line L3828 (224.18, 23.934) -> (238.182, 23.934)
  line L3829 (-127.7325, 19.8345) -> (-128.5329, 19.8345)
  line L3830 (13.831, 108.6602) -> (14.63, 108.6602)
  line L3831 (-128.2451, 68.0838) -> (-129.0441, 68.0838)
  line L3832 (-124.283, 22.9336) -> (-123.4826, 22.9336)
  line L3833 (-128.2451, 71.1844) -> (-128.2451, 76.9844)
  line L3834 (238.979, 10.9337) -> (238.182, 10.9337)
  line L3835 (-5.219, 108.6602) -> (-5.219, 105.5592)
  line L3836 (-128.2451, 68.0838) -> (-128.2451, 67.0833)
  line L3837 (29.43, 108.6602) -> (28.631, 108.6602)
  line L3838 (238.979, 14.0343) -> (238.979, 10.9337)
  line L3839 (-163.9637, -5.0157) -> (-163.9637, 0.7845)
  line L3840 (258.029, 71.1844) -> (258.029, 68.0838)
  line L3841 (-109.4829, 22.9336) -> (-109.4829, 23.934)
  line L3842 (-129.0441, 76.9844) -> (-128.2451, 76.9844)
  line L3843 (242.482, 17.6585) -> (243.459, 17.6585)
  line L3844 (-4.42, 96.6592) -> (-4.42, 95.6582)
  line L3845 (19.106, 67.0833) -> (5.105, 67.0833)
  line L3846 (-123.4826, 19.8345) -> (-123.4826, 14.0343)
  line L3847 (28.631, 109.6602) -> (14.63, 109.6602)
  line L3848 (-149.9629, -5.0157) -> (-149.9629, 0.7845)
  line L3849 (238.182, 68.0838) -> (238.182, 67.0833)
  line L3850 (-149.9629, 19.8345) -> (-149.9629, 14.0343)
  line L3851 (-8.67, 99.7592) -> (-8.67, 96.6592)
  line L3852 (-127.7325, 22.9336) -> (-128.5329, 22.9336)
  line L3853 (243.23, 0.4083) -> (243.23, 14.4091)
  line L3854 (-128.2451, 67.0833) -> (-114.244, 67.0833)
  line L3855 (244.232, 15.2084) -> (244.232, 14.4091)
  line L3856 (238.979, 68.0838) -> (238.979, 71.1844)
  line L3857 (-149.1636, -5.0157) -> (-149.1636, -8.1163)
  line L3858 (243.23, 14.4091) -> (243.23, 0.4083)
  line L3859 (-4.42, 108.6602) -> (-4.42, 109.6602)
  line L3860 (242.429, 71.1844) -> (243.23, 71.1844)
  line L3861 (-42.808, 42.984) -> (-56.808, 42.984)
  line L3862 (-4.42, 105.5592) -> (-5.219, 105.5592)
  line L3863 (9.581, 109.6602) -> (-4.42, 109.6602)
  line L3864 (14.63, 105.5592) -> (14.63, 99.7592)
  line L3865 (238.182, 48.0333) -> (224.18, 48.0333)
  line L3866 (-163.9637, 0.7845) -> (-163.9637, -5.0157)
  line L3867 (-8.67, 108.6602) -> (-8.67, 105.5592)
  line L3868 (224.18, 48.0333) -> (238.182, 48.0333)
  line L3869 (-127.7325, 19.8345) -> (-127.7325, 22.9336)
  line L3870 (-61.57, 57.9344) -> (-61.57, 52.1344)
  line L3871 (243.459, 15.9333) -> (243.459, 17.6585)
  line L3872 (257.232, 0.4083) -> (257.232, 14.4091)
  line L3873 (-61.57, 62.034) -> (-47.569, 62.034)
  line L3874 (-62.371, 61.0336) -> (-62.371, 57.9344)
  line L3875 (-133.294, 71.1844) -> (-133.294, 76.9844)
  line L3876 (-128.5329, 23.934) -> (-128.5329, 22.9336)
  line L3877 (-133.294, 68.0838) -> (-132.495, 68.0838)
  line L3878 (257.232, 14.4091) -> (257.232, 0.4083)
  line L3879 (247.929, 15.9333) -> (247.929, 14.4091)
  line L3880 (-163.9637, -9.1167) -> (-163.9637, -8.1163)
  line L3881 (-163.9637, -5.0157) -> (-164.763, -5.0157)
  line L3882 (-37.758, 38.8844) -> (-37.758, 33.0844)
  line L3883 (238.979, 10.9337) -> (238.979, 14.0343)
  line L3884 (-62.371, 52.1344) -> (-62.371, 49.0338)
  line L3885 (-38.558, 33.0844) -> (-38.558, 29.9838)
  line L3886 (-4.42, 96.6592) -> (-5.219, 96.6592)
  line L3887 (14.63, 99.7592) -> (14.63, 105.5592)
  line L3888 (238.182, 14.0343) -> (238.182, 19.8345)
  line L3889 (-38.044, 67.0833) -> (-52.045, 67.0833)
  line L3890 (-8.67, 96.6592) -> (-8.67, 99.7592)
  line L3891 (-128.2451, 76.9844) -> (-128.2451, 71.1844)
  line L3892 (-4.42, 52.1344) -> (-5.219, 52.1344)
  line L3893 (-108.6825, 19.8345) -> (-109.4829, 19.8345)
  line L3894 (-128.2451, 80.0836) -> (-128.2451, 81.084)
  line L3895 (-164.763, -5.0157) -> (-163.9637, -5.0157)
  line L3896 (-124.283, 19.8345) -> (-123.4826, 19.8345)
  line L3897 (-37.758, 29.9838) -> (-38.558, 29.9838)
  line L3898 (-149.1636, 0.7845) -> (-149.1636, 3.8837)
  line L3899 (-164.763, 0.7845) -> (-164.763, 3.8837)
  line L3900 (244.232, 15.2084) -> (247.333, 15.2084)
  line L3901 (-109.4829, 23.934) -> (-109.4829, 22.9336)
  line L3902 (-4.42, 61.0336) -> (-4.42, 62.034)
  line L3903 (-42.007, 38.8844) -> (-42.007, 41.9836)
  line L3904 (-62.371, 57.9344) -> (-62.371, 61.0336)
  line L3905 (-38.558, 33.0844) -> (-37.758, 33.0844)
  line L3906 (-4.42, 95.6582) -> (-4.42, 96.6592)
  line L3907 (-4.42, 109.6602) -> (-4.42, 108.6602)
  line L3908 (-62.371, 61.0336) -> (-61.57, 61.0336)
  line L3909 (-149.9629, -9.1167) -> (-163.9637, -9.1167)
  line L3910 (-5.219, 99.7592) -> (-5.219, 96.6592)
  line L3911 (-5.219, 57.9344) -> (-5.219, 61.0336)
  line L3912 (-163.9637, 0.7845) -> (-164.763, 0.7845)
  line L3913 (-128.5329, 14.0343) -> (-128.5329, 19.8345)
  line L3914 (-4.42, 49.0338) -> (-5.219, 49.0338)
  line L3915 (-5.219, 105.5592) -> (-5.219, 108.6602)
  line L3916 (-113.9576, 28.9833) -> (-99.9579, 28.9833)
  line L3917 (238.182, 14.0343) -> (238.979, 14.0343)
  line L3918 (-37.758, 42.984) -> (-37.758, 41.9836)
  line L3919 (-47.569, 62.034) -> (-61.57, 62.034)
  line L3920 (-62.371, 49.0338) -> (-62.371, 52.1344)
  line L3921 (-123.4826, 22.9336) -> (-123.4826, 23.934)
  line L3922 (-164.763, 3.8837) -> (-164.763, 0.7845)
  line L3923 (-149.1636, -8.1163) -> (-149.9629, -8.1163)
  line L3924 (247.929, 14.4091) -> (247.333, 14.4091)
  line L3925 (-149.9629, -8.1163) -> (-149.1636, -8.1163)
  line L3926 (-61.57, 61.0336) -> (-61.57, 62.034)
  line L3927 (238.979, 14.0343) -> (238.182, 14.0343)
  line L3928 (-42.007, 33.0844) -> (-42.007, 29.9838)
  line L3929 (-37.758, 41.9836) -> (-38.558, 41.9836)
  circle A63 centre (19.098, 117.5832) radius 1.7
  line L3930 (238.182, 10.9337) -> (238.979, 10.9337)
  line L3931 (-113.9576, 42.984) -> (-99.9579, 42.984)
  line L3932 (-164.763, -8.1163) -> (-164.763, -5.0157)
  line L3933 (-62.371, 57.9344) -> (-61.57, 57.9344)
  line L3934 (-5.219, 105.5592) -> (-4.42, 105.5592)
  line L3935 (-99.9579, 42.984) -> (-113.9576, 42.984)
  line L3936 (-38.558, 38.8844) -> (-37.758, 38.8844)
  line L3937 (243.459, 15.9333) -> (247.929, 15.9333)
  line L3938 (29.43, 108.6602) -> (29.43, 105.5592)
  line L3939 (-4.42, 48.0333) -> (-4.42, 49.0338)
  line L3940 (-8.67, 105.5592) -> (-8.67, 108.6602)
  line L3941 (14.63, 109.6602) -> (14.63, 108.6602)
  line L3942 (-5.219, 108.6602) -> (-4.42, 108.6602)
  line L3943 (-99.9579, 28.9833) -> (-113.9576, 28.9833)
  line L3944 (-37.758, 33.0844) -> (-38.558, 33.0844)
  line L3945 (28.631, 105.5592) -> (29.43, 105.5592)
  line L3946 (-38.558, 29.9838) -> (-38.558, 33.0844)
  line L3947 (-56.808, 42.984) -> (-42.808, 42.984)
  line L3948 (-4.42, 52.1344) -> (-4.42, 57.9344)
  line L3949 (-163.9637, -9.1167) -> (-149.9629, -9.1167)
  line L3950 (-5.219, 61.0336) -> (-4.42, 61.0336)
  line L3951 (243.459, 17.6585) -> (242.482, 17.6585)
  line L3952 (-61.57, 49.0338) -> (-61.57, 48.0333)
  line L3953 (243.459, 17.6585) -> (243.459, 15.9333)
  line L3954 (-149.1636, 3.8837) -> (-149.1636, 0.7845)
  line L3955 (-61.57, 62.034) -> (-61.57, 61.0336)
  line L3956 (29.43, 105.5592) -> (29.43, 108.6602)
  line L3957 (-4.42, 108.6602) -> (-5.219, 108.6602)
  line L3958 (-37.758, 38.8844) -> (-38.558, 38.8844)
  line L3959 (-61.57, 49.0338) -> (-62.371, 49.0338)
  line L3960 (244.232, 14.4091) -> (244.232, 15.2084)
  line L3961 (-62.371, 49.0338) -> (-61.57, 49.0338)
  line L3962 (14.63, 108.6602) -> (14.63, 109.6602)
  line L3963 (-4.42, 99.7592) -> (-4.42, 105.5592)
  line L3964 (-5.219, 49.0338) -> (-4.42, 49.0338)
  line L3965 (-9.469, 105.5592) -> (-9.469, 99.7592)
  line L3966 (238.182, 9.9333) -> (238.182, 10.9337)
  line L3967 (-37.758, 41.9836) -> (-37.758, 42.984)
  line L3968 (-9.469, 99.7592) -> (-8.67, 99.7592)
  line L3969 (13.831, 105.5592) -> (14.63, 105.5592)
  line L3970 (-5.219, 61.0336) -> (-5.219, 57.9344)
  line L3971 (-38.558, 41.9836) -> (-37.758, 41.9836)
  line L3972 (-61.57, 57.9344) -> (-62.371, 57.9344)
  line L3973 (-8.67, 96.6592) -> (-9.469, 96.6592)
  line L3974 (253.129, 15.2084) -> (253.129, 14.4091)
  line L3975 (-61.57, 48.0333) -> (-61.57, 49.0338)
  line L3976 (247.929, 15.9333) -> (243.459, 15.9333)
  line L3977 (238.182, 19.8345) -> (238.182, 14.0343)
  line L3978 (13.831, 105.5592) -> (13.831, 108.6602)
  line L3979 (-4.42, 49.0338) -> (-4.42, 48.0333)
  line L3980 (-61.57, 61.0336) -> (-62.371, 61.0336)
  line L3981 (-61.57, 52.1344) -> (-61.57, 57.9344)
  line L3982 (256.681, 17.6585) -> (255.761, 17.6585)
  line L3983 (-5.219, 52.1344) -> (-5.219, 49.0338)
  line L3984 (256.23, 14.4091) -> (256.23, 15.2084)
  line L3985 (-38.558, 38.8844) -> (-38.558, 41.9836)
  line L3986 (-9.469, 96.6592) -> (-9.469, 95.6582)
  line L3987 (257.232, 14.4091) -> (256.23, 14.4091)
  line L3988 (-5.219, 57.9344) -> (-4.42, 57.9344)
  line L3989 (-62.371, 52.1344) -> (-61.57, 52.1344)
  line L3990 (-56.295, 71.1844) -> (-56.295, 68.0838)
  line L3991 (-65.82, 61.0336) -> (-66.62, 61.0336)
  line L3992 (-151.5449, 68.0838) -> (-151.5449, 71.1844)
  line L3993 (-151.5449, 99.7592) -> (-151.5449, 96.6592)
  line L3994 (-32.482, 22.9336) -> (-33.283, 22.9336)
  line L3995 (-52.844, 68.0838) -> (-52.844, 71.1844)
  line L3996 (-47.283, 23.934) -> (-33.283, 23.934)
  line L3997 (-56.295, 76.9844) -> (-57.094, 76.9844)
  line L3998 (-91.2764, 3.4138) -> (-89.551, 3.4138)
  line L3999 (-51.532, 22.9336) -> (-52.333, 22.9336)
  line L4000 (255.761, -2.8412) -> (256.681, -2.8412)
  line L4001 (-148.0943, 80.0836) -> (-147.295, 80.0836)
  line L4002 (249.732, -8.6909) -> (252.529, -8.6909)
  line L4003 (-92.1019, -2.6165) -> (-92.1019, 0.1836)
  line L4004 (-102.3378, 3.8837) -> (-101.5387, 3.8837)
  line L4005 (-52.045, 68.0838) -> (-52.045, 67.0833)
  line L4006 (-148.0943, 76.9844) -> (-148.0943, 80.0836)
  line L4007 (-147.295, 71.1844) -> (-147.295, 76.9844)
  line L4008 (-148.0943, 71.1844) -> (-148.0943, 68.0838)
  line L4009 (255.761, -1.1159) -> (252.529, -1.1159)
  line L4010 (256.23, -0.391) -> (256.23, 0.4083)
  line L4011 (0.056, 80.0836) -> (0.056, 81.084)
  line L4012 (-33.283, 23.934) -> (-47.283, 23.934)
  line L4013 (-147.295, 68.0838) -> (-147.295, 67.0833)
  line L4014 (-92.1019, 0.1836) -> (-91.2764, 0.1836)
  line L4015 (-57.094, 71.1844) -> (-56.295, 71.1844)
  line L4016 (247.333, -0.391) -> (247.333, 0.4083)
  line L4017 (-102.3378, 0.7845) -> (-102.3378, -5.0157)
  line L4018 (-57.094, 71.1844) -> (-57.094, 76.9844)
  line L4019 (-52.045, 71.1844) -> (-52.045, 76.9844)
  line L4020 (-48.083, 19.8345) -> (-48.083, 22.9336)
  line L4021 (-101.5387, -8.1163) -> (-102.3378, -8.1163)
  line L4022 (-152.3441, 108.6602) -> (-151.5449, 108.6602)
  line L4023 (-71.8941, 71.1844) -> (-71.8941, 68.0838)
  line L4024 (-147.295, 80.0836) -> (-147.295, 81.084)
  line L4025 (-47.283, 22.9336) -> (-47.283, 23.934)
  line L4026 (-65.82, 49.0338) -> (-65.82, 52.1344)
  line L4027 (-65.82, 49.0338) -> (-66.62, 49.0338)
  line L4028 (-57.094, 80.0836) -> (-56.295, 80.0836)
  line L4029 (-76.144, 76.9844) -> (-75.345, 76.9844)
  line L4030 (247.929, -1.1159) -> (247.929, 0.4083)
  line L4031 (255.761, -6.1416) -> (255.761, -7.8669)
  line L4032 (-32.482, 19.8345) -> (-33.283, 19.8345)
  arc A64 (-145.2635, 118.9832) -> (-147.2635, 120.9832) centre (-147.2635, 118.9832) ccw
  line L4033 (-71.8941, 80.0836) -> (-71.8941, 76.9844)
  line L4034 (-65.82, 61.0336) -> (-65.82, 57.9344)
  line L4035 (-56.295, 80.0836) -> (-56.295, 76.9844)
  line L4036 (-152.3441, 99.7592) -> (-151.5449, 99.7592)
  line L4037 (-91.2764, 0.1836) -> (-91.2764, 3.4138)
  line L4038 (-66.62, 57.9344) -> (-66.62, 52.1344)
  line L4039 (-89.551, 3.4138) -> (-91.2764, 3.4138)
  line L4040 (-48.083, 19.8345) -> (-47.283, 19.8345)
  line L4041 (-148.0943, 80.0836) -> (-148.0943, 76.9844)
  line L4042 (-52.045, 67.0833) -> (-52.045, 68.0838)
  line L4043 (-71.095, 81.084) -> (-71.095, 80.0836)
  line L4044 (-33.283, 23.934) -> (-33.283, 22.9336)
  line L4045 (253.129, 0.4083) -> (253.129, -0.391)
  line L4046 (-152.3441, 99.7592) -> (-152.3441, 105.5592)
  line L4047 (255.761, -7.8669) -> (252.529, -7.8669)
  line L4048 (252.529, -7.8669) -> (252.529, -8.6909)
  line L4049 (-148.0943, 68.0838) -> (-148.0943, 71.1844)
  line L4050 (-108.6825, 14.0343) -> (-109.4829, 14.0343)
  line L4051 (-57.094, 68.0838) -> (-56.295, 68.0838)
  line L4052 (-101.5387, -5.0157) -> (-101.5387, -8.1163)
  line L4053 (-91.2764, -2.6165) -> (-91.2764, -8.8866)
  line L4054 (-65.82, 52.1344) -> (-65.82, 49.0338)
  line L4055 (-71.095, 76.9844) -> (-71.095, 71.1844)
  line L4056 (-108.6825, 10.9337) -> (-109.4829, 10.9337)
  line L4057 (-109.4829, 14.0343) -> (-108.6825, 14.0343)
  line L4058 (252.529, -8.6909) -> (249.732, -8.6909)
  line L4059 (256.681, -6.1416) -> (255.761, -6.1416)
  line L4060 (-75.345, 80.0836) -> (-76.144, 80.0836)
  line L4061 (-61.057, 41.9836) -> (-61.057, 38.8844)
  line L4062 (-108.6825, 14.0343) -> (-108.6825, 10.9337)
  line L4063 (253.129, 0.4083) -> (252.529, 0.4083)
  line L4064 (-47.283, 22.9336) -> (-48.083, 22.9336)
  line L4065 (-71.095, 67.0833) -> (-71.095, 68.0838)
  line L4066 (-65.82, 57.9344) -> (-66.62, 57.9344)
  line L4067 (-91.2764, -8.8866) -> (-91.2764, -2.6165)
  line L4068 (-148.0943, 76.9844) -> (-147.295, 76.9844)
  line L4069 (-147.295, 80.0836) -> (-148.0943, 80.0836)
  line L4070 (-56.808, 42.984) -> (-56.808, 41.9836)